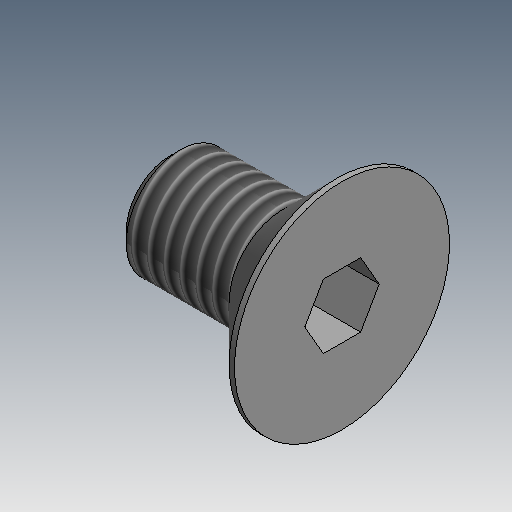
# Autodesk Inventor part: FB10-16_
Saved by Autodesk Inventor 2020 (Build 240168000, 168)
## iProperties
Part Number: FB10-16_
Material: 一般
Catalog Web Link: www.cadenas.de
Description: FB_-Hexagon Socket Head Cap Screws
Vendor: MISUMI
Document SubType Name: Modeling
Designer: partserver
Manufacturer: MISUMI
Mass: 1.74081 g
Surface Area: 11.6162 cm^2
Volume: 1.74081 cm^3
Density: 1 g/cm^3
Appearance: PSOLRGB-192-192-192
Category: PARTsolutions
Company: MISUMI
PSOL_IDENT_0: {$CADENAS_DATA\23d-libs\misumi\metric\38_al_extrusions_blackets\fb_.prj},156 {VTYP=3D},{NB=FB10-16_}
PSOL_IDENT_1: ,{LINA=FB10-16_},{NN=FB_},{DATE=30.06.2021 13:17:46},{GEOMDATE=31.03.2009 00:00:00},{VERSION=},{LINE
PSOL_IDENT_2: ID=100},{WBVAR=L},{WBNUMERIC=L}  {NB=FB10-16_},{LINA=FB10-16_},{KT=DUMMY},{PN=FB10-16_},{MAT=4137 St
PSOL_IDENT_3: eel},{HARD=32~38HRC},{M=10},{L=16},{LL=Full Thread},{L1=22},{TYPE=FB},{L0=16,20},{NDM=10},{KDM=8.156
PSOL_IDENT_4: 995},{MP=10x1.5},{P=1.5},{A=20},{E=5.5},{B=6.0}
NB: FB10-16_
NN: FB_
NT: Hexagon Socket Head Cap Screws
NBSYN: $PN.
LINA: FB10-16_
CATALOG: Misumi
PN: FB10-16_
MAT: 4137 Steel
HARD: 32~38HRC
M: 10
L: 16
LL: Full Thread
MP: 10x1.5
A: 20
E: 5.5
B: 6
SUPPLIER: MISUMI
ARTICLENO: FB10-16_
BOMINFO: FB10-16_
CREATOR: CADENAS GmbH
d12: 0.000 mm
Title: FB10-16_
Author: Cadenas PARTsolutions
Comments: Hexagon Socket Head Cap Screws
Autodesk Inventor part; units mm, degrees
sketch "Sketch_1" plane through (0, 0, 0) normal (0, 0, 1) x (1, 0, 0)
  line L0 (16, 0) -> (0, 0)
  line L1 (0, 0) -> (0, 10)
  line L2 (0, 10) -> (0.5, 10)
  line L3 (0.5, 10) -> (5.5, 5)
  line L4 (5.5, 5) -> (15.08, 5)
  line L5 (15.08, 5) -> (16, 4.08)
  line L6 (16, 4.08) -> (16, 0)
  line L7 (16, 0) -> (0, 0)
  constraints: 16 end point
revolve "Revolution1" add sketch "Sketch_1" angle 360 about axis through (16, 0, 0) along (1, 0, 0)
thread "Thread1" size "M10x1.5" class "6g" standard "ISO Metric profile" full length
sketch "Sketch2" plane through (0, 0, 0) normal (-1, 0, 0) x (0, 0, 1)
  point P0 (0, 0)
hole "Hole1" at (0, 0, 0) direction (1, 0, 0) diameter 6 depth 4.4 tip angle 150
sketch "Sketch_3" plane through (0, 0, 0) normal (1, 0, 0) x (0, 1, 0)
  line L0 (-1.7321, 3) -> (-3.4641, 0)
  line L1 (-3.4641, 0) -> (-1.7321, -3)
  line L2 (-1.7321, -3) -> (1.7321, -3)
  line L3 (1.7321, -3) -> (3.4641, 0)
  line L4 (3.4641, 0) -> (1.7321, 3)
  line L5 (1.7321, 3) -> (-1.7321, 3)
  constraints: 12 end point
extrude "Extrusion1" cut sketch "Sketch_3" along normal blind 4.4
ref_plane "screw_to_nut_XY" through (0, 0, 0) normal (1, 0, 0) x (0, 0, -1)
ref_plane "screw_to_nut_YZ" through (0, 0, 0) normal (0, 0, -1) x (0, 1, 0)
ref_plane "screw_to_nut_ZX" through (0, 0, 0) normal (0, 1, 0) x (1, 0, 0)
body "Solid1"
